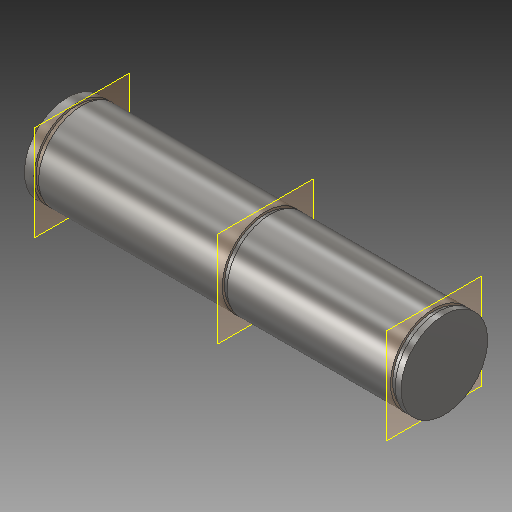
# Autodesk Inventor part: Shaft-2
Saved by Autodesk Inventor 2019.4 (Build 234330000, 330)
## iProperties
Created: 2020-01-06
Part Number: Shaft-2
Material: Steel, Alloy
Document SubType Name: Modeling
Designer: Mark
Mass: 211.275 g
Surface Area: 60.9469 cm^2
Volume: 27.3319 cm^3
Density: 7.73 g/cm^3
Appearance: Semi-Polished
Author: Mark
Autodesk Inventor part; units mm, degrees
ref_plane "YZ Plane" through (0, 0, 0) normal (1, 0, 0) x (0, 1, 0)
ref_plane "XZ Plane" through (0, 0, 0) normal (0, 1, 0) x (-1, 0, 0)
ref_plane "XY Plane" through (0, 0, 0) normal (0, 0, 1) x (1, 0, 0)
sketch "Sketch1" plane through (0, 0, 0) normal (1, 0, 0) x (0, 1, 0)
  circle A0 centre (0, 0) radius 10
  dimension "d0" = 20
  constraints: 1 centre point, 1 coincident
  measures "d0" diameter of A0
extrude "Extrusion1" add sketch "Sketch1" along normal blind 87
ref_plane "Work Plane1" through (84.551, 0, 0) normal (1, 0, 0) x (0, 0, -1)
sketch "Sketch2" plane through (84.551, 0, 0) normal (1, 0, 0) x (0, 0, -1)
  circle A0 centre (0, 0) radius 9.5
  circle A1 centre (0, 0) radius 10.5
  dimension "d4" = 19
  dimension "d5" = 21
  constraints: 2 centre point, 2 coincident
  measures "d4" diameter of A0
  measures "d5" diameter of A1
extrude "Extrusion2" cut sketch "Sketch2" along normal blind 1.1
ref_plane "Work Plane2" through (45.7, 0, 0) normal (1, 0, 0) x (0, 0, -1)
sketch "Sketch3" plane through (45.7, 0, 0) normal (1, 0, 0) x (0, 0, -1)
  circle A0 centre (0, 0) radius 9.5
  circle A1 centre (0, 0) radius 10.5
  dimension "d9" = 19
  dimension "d10" = 21
  constraints: 2 centre point, 2 coincident
  measures "d9" diameter of A0
  measures "d10" diameter of A1
extrude "Extrusion3" cut sketch "Sketch3" along normal blind 1.1
ref_plane "Work Plane3" through (3.3, 0, 0) normal (1, 0, 0) x (0, 0, -1)
sketch "Sketch4" plane through (3.3, 0, 0) normal (1, 0, 0) x (0, 0, -1)
  circle A0 centre (0, 0) radius 9.5
  circle A1 centre (0, 0) radius 10.5
  dimension "d14" = 19
  dimension "d15" = 21
  constraints: 2 centre point, 2 coincident
  measures "d14" diameter of A0
  measures "d15" diameter of A1
extrude "Extrusion4" cut sketch "Sketch4" against normal blind 1.1
body "Solid1"
